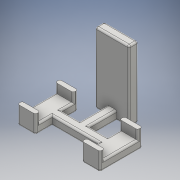
# Autodesk Inventor part: handle
Saved by Autodesk Inventor 2016 (Build 200138000, 138)
## iProperties
Created: 2016-05-24
Part Number: handle
Material: ABS Plastic
Document SubType Name: Modeling
Designer: Hamid Osooli
Density: 1.06 g/cm^3
Appearance: Smooth - White
Mass: 50.8202 g
Surface Area: 188.654 cm^2
Volume: 47.9436 cm^3
Author: Hamid Osooli
Autodesk Inventor part; units mm, degrees
ref_plane "YZ Plane" through (0, 0, 0) normal (1, 0, 0) x (0, 1, 0)
ref_plane "XZ Plane" through (0, 0, 0) normal (0, 1, 0) x (-1, 0, 0)
ref_plane "XY Plane" through (0, 0, 0) normal (0, 0, 1) x (1, 0, 0)
sketch "Sketch1" plane through (0, 0, 0) normal (0, 0, 1) x (1, 0, 0)
  line L0 (42.75, 23) -> (27.25, 23)
  line L1 (25.25, 21) -> (25.25, 20)
  line L2 (27.25, 18) -> (42.75, 18)
  line L3 (44.75, 20) -> (44.75, 21)
  line L4 (-42.75, 23) -> (-27.25, 23)
  line L5 (-25.25, 21) -> (-25.25, 20)
  line L6 (-27.25, 18) -> (-42.75, 18)
  line L7 (-44.75, 20) -> (-44.75, 21)
  line L8 (42.75, -23) -> (27.25, -23)
  line L9 (25.25, -21) -> (25.25, -20)
  line L10 (27.25, -18) -> (42.75, -18)
  line L11 (44.75, -20) -> (44.75, -21)
  line L12 (-42.75, -23) -> (-27.25, -23)
  line L13 (-25.25, -21) -> (-25.25, -20)
  line L14 (-27.25, -18) -> (-42.75, -18)
  line L15 (-44.75, -20) -> (-44.75, -21)
  arc A0 (44.75, 21) -> (42.75, 23) centre (42.75, 21) ccw
  arc A1 (42.75, 18) -> (44.75, 20) centre (42.75, 20) ccw
  arc A2 (25.25, 20) -> (27.25, 18) centre (27.25, 20) ccw
  arc A3 (27.25, 23) -> (25.25, 21) centre (27.25, 21) ccw
  arc A4 (44.75, -20) -> (42.75, -18) centre (42.75, -20) ccw
  arc A5 (42.75, -23) -> (44.75, -21) centre (42.75, -21) ccw
  arc A6 (25.25, -21) -> (27.25, -23) centre (27.25, -21) ccw
  arc A7 (27.25, -18) -> (25.25, -20) centre (27.25, -20) ccw
  arc A8 (-25.25, 21) -> (-27.25, 23) centre (-27.25, 21) ccw
  arc A9 (-27.25, 18) -> (-25.25, 20) centre (-27.25, 20) ccw
  arc A10 (-44.75, 20) -> (-42.75, 18) centre (-42.75, 20) ccw
  arc A11 (-42.75, 23) -> (-44.75, 21) centre (-42.75, 21) ccw
  arc A12 (-25.25, -20) -> (-27.25, -18) centre (-27.25, -20) ccw
  arc A13 (-27.25, -23) -> (-25.25, -21) centre (-27.25, -21) ccw
  arc A14 (-44.75, -21) -> (-42.75, -23) centre (-42.75, -21) ccw
  arc A15 (-42.75, -18) -> (-44.75, -20) centre (-42.75, -20) ccw
  point P0 (25.25, 18)
  point P1 (44.75, 18)
  point P2 (-25.25, 18)
  point P3 (-44.75, 18)
  point P4 (25.25, -18)
  point P5 (44.75, -18)
  point P6 (-25.25, -18)
  point P7 (-44.75, -18)
  dimension "d86" = 19.5
  dimension "d88" = 19.5
  dimension "d90" = 19.5
  dimension "d92" = 19.5
  dimension "d94" = 2
  dimension "d95" = 2
  constraints: 32 end point, 32 point on circle, 32 tangent, 16 centre point, 16 point on line, 14 equal radius, 8 parallel, 4 horizontal, 4 perpendicular
  measures "d86" distance of point (44.75, 18) point (25.25, 18)
  measures "d88" distance of point (-25.25, 18) point (-44.75, 18)
  measures "d90" distance of point (25.25, -18) point (44.75, -18)
  measures "d92" distance of point (-44.75, -18) point (-25.25, -18)
  measures "d94" radius of A0
  measures "d95" radius of A8
extrude "Extrusion1" add sketch "Sketch1" along normal blind 10
sketch "Sketch2" plane through (0, 0, 0) normal (0, 0, 1) x (1, 0, 0)
  line L0 (-42.75, 23) -> (-27.25, 23)
  line L1 (-25.25, 21) -> (-25.25, -21)
  line L2 (-27.25, -23) -> (-42.75, -23)
  line L3 (-44.75, -21) -> (-44.75, 21)
  line L4 (42.75, 23) -> (27.25, 23)
  line L5 (25.25, 21) -> (25.25, -21)
  line L6 (27.25, -23) -> (42.75, -23)
  line L7 (44.75, -21) -> (44.75, 21)
  arc A0 (-42.75, 23) -> (-44.75, 21) centre (-42.75, 21) ccw
  arc A1 (-25.25, 21) -> (-27.25, 23) centre (-27.25, 21) ccw
  arc A2 (-27.25, -23) -> (-25.25, -21) centre (-27.25, -21) ccw
  arc A3 (-44.75, -21) -> (-42.75, -23) centre (-42.75, -21) ccw
  arc A4 (25.25, -21) -> (27.25, -23) centre (27.25, -21) ccw
  arc A5 (42.75, -23) -> (44.75, -21) centre (42.75, -21) ccw
  arc A6 (44.75, 21) -> (42.75, 23) centre (42.75, 21) ccw
  arc A7 (27.25, 23) -> (25.25, 21) centre (27.25, 21) ccw
  point P0 (0, 0)
  point P1 (-25.25, -23)
  point P2 (-25.25, 23)
  point P3 (-44.75, -23)
  point P4 (25.25, -23)
  point P5 (25.25, 23)
  point P6 (44.75, -23)
  dimension "d96" = 19.5
  dimension "d97" = 46
  dimension "d98" = 19.5
  dimension "d99" = 46
  dimension "d100" = 2
  constraints: 16 end point, 16 point on circle, 16 tangent, 12 point on line, 8 centre point, 7 equal radius, 4 parallel, 2 horizontal, 2 perpendicular
  measures "d96" distance of point (-25.25, -23) point (-44.75, -23)
  measures "d97" distance of point (-25.25, 23) point (-25.25, -23)
  measures "d98" distance of point (44.75, -23) point (25.25, -23)
  measures "d99" distance of point (25.25, -23) point (25.25, 23)
  measures "d100" radius of A0
extrude "Extrusion2" add sketch "Sketch2" against normal blind 10
sketch "Sketch9" plane through (25.25, -20, 0) normal (-1, 0, 0) x (0, 0, 1)
  line L0 (0, 0) -> (0, 40) projected
  line L1 (-10, -1) -> (-10, 41) projected
  line L2 (0, 25) -> (-10, 25)
  line L3 (-10, 25) -> (-10, 15)
  line L4 (-10, 15) -> (0, 15)
  line L5 (0, 15) -> (0, 25)
  point P0 (0, 20)
  dimension "d101" = 10
  constraints: 8 end point, 2 parallel, 2 point on line, 1 horizontal, 1 perpendicular
  measures "d101" distance of L3.end L2.end
extrude "Extrusion9" add sketch "Sketch9" along normal up to next
sketch "Sketch12" plane through (0, 0, -10) normal (0, 0, -1) x (-1, 0, 0)
  line L0 (18.5, 35) -> (-18.5, 35)
  line L1 (-18.5, 35) -> (-18.5, 45)
  line L2 (-18.5, 45) -> (18.5, 45)
  line L3 (18.5, 45) -> (18.5, 35)
  point P0 (0, 0)
  dimension "d108" = 37
  dimension "d109" = 10
  constraints: 8 end point, 2 parallel, 1 horizontal, 1 perpendicular
  measures "d108" distance of L1.end L2.end
  measures "d109" distance of L0.end L1.end
extrude "Extrusion11" add sketch "Sketch12" against normal blind 77
sketch "Sketch14" plane through (-18.5, 45, -10) normal (0, 1, 0) x (1, 0, 0)
  line L0 (6.75, -5) -> (30.25, -5)
  line L1 (32.25, -7) -> (32.25, -70)
  line L2 (30.25, -72) -> (6.75, -72)
  line L3 (4.75, -70) -> (4.75, -7)
  arc A0 (6.75, -5) -> (4.75, -7) centre (6.75, -7) ccw
  arc A1 (32.25, -7) -> (30.25, -5) centre (30.25, -7) ccw
  arc A2 (30.25, -72) -> (32.25, -70) centre (30.25, -70) ccw
  arc A3 (4.75, -70) -> (6.75, -72) centre (6.75, -70) ccw
  point P0 (32.25, -72)
  point P1 (32.25, -5)
  point P2 (4.75, -72)
  dimension "d112" = 27.5
  dimension "d113" = 67
  dimension "d114" = 2
  constraints: 8 end point, 8 point on circle, 8 tangent, 6 point on line, 4 centre point, 3 equal radius, 2 parallel, 1 horizontal, 1 perpendicular
  measures "d112" distance of point (32.25, -72) point (4.75, -72)
  measures "d113" distance of point (32.25, -5) point (32.25, -72)
  measures "d114" radius of A0
extrude "Extrusion12" cut sketch "Sketch14" against normal blind 5
sketch "Sketch15" plane through (-18.5, 40, -10) normal (0, 1, 0) x (1, 0, 0)
  circle A0 centre (9.5, -8.5) radius 1.75
  circle A1 centre (27.5, -8.5) radius 1.75
  circle A2 centre (27.5, -68.5) radius 1.75
  circle A3 centre (9.5, -68.5) radius 1.75
  point P0 (18.5, -10)
  dimension "d125" = 3.5
  dimension "d126" = 3.5
  dimension "d127" = 3.5
  dimension "d128" = 3.5
  constraints: 4 centre point
  measures "d125" diameter of A0
  measures "d126" diameter of A1
  measures "d127" diameter of A2
  measures "d128" diameter of A3
extrude "Extrusion13" add sketch "Sketch15" along normal blind 5
sketch "Sketch17" plane through (25.25, 5, 0) normal (0, 1, 0) x (1, 0, 0)
  line L0 (0, 0) -> (-50.5, 0) projected
  line L1 (-30.25, 0) -> (-20.25, 0)
  line L2 (-20.25, 0) -> (-20.25, 10)
  line L3 (-20.25, 10) -> (-30.25, 10)
  line L4 (-30.25, 10) -> (-30.25, 0)
  point P0 (-25.25, 0)
  dimension "d134" = 10
  dimension "d135" = 10
  constraints: 8 end point, 2 parallel, 1 horizontal, 1 perpendicular, 1 point on line
  measures "d134" distance of L3.end L2.end
  measures "d135" distance of L2.end L1.end
extrude "Extrusion15" add sketch "Sketch17" along normal up to next
sketch "Sketch19" plane through (-18.5, 45, -10) normal (0, 1, 0) x (1, 0, 0)
  line L0 (23.5, 0) -> (23.5, -10) projected
  line L1 (13.5, -10) -> (13.5, 0) projected
  line L2 (23.5, -5) -> (13.5, -5)
  line L3 (13.5, -5) -> (13.5, 0)
  line L4 (13.5, 0) -> (23.5, 0)
  line L5 (23.5, 0) -> (23.5, -5)
  point P0 (18.5, -10)
  dimension "d138" = 10
  constraints: 8 end point, 2 parallel, 1 horizontal, 1 midpoint, 1 perpendicular
  measures "d138" distance of L1.end L4.end
extrude "Extrusion16" cut sketch "Sketch19" against normal blind 5
fillet "Fillet5" radius 2 14 edges at (18.5, 45, 28.5) (11.75, 45, -10) (11.75, 35, -10) (18.5, 40, -10) (-11.75, 45, -10) (-11.75, 35, -10) (-18.5, 40, -10) (-18.5, 45, 28.5) (-18.5, 35, 28.5) (-18.5, 40, 67) (0, 35, 67) (18.5, 40, 67) (0, 45, 67) (18.5, 35, 28.5)
fillet "Fillet6" radius 2 24 edges at (-25.8358, 22.4142, -10) (-35, 23, -10) (-44.1642, 22.4142, -10) (-44.75, 0, -10) (-44.1642, -22.4142, -10) (-35, -23, -10) (-25.8358, -22.4142, -10) (-25.25, -13, -10) (-25.25, 13, -10) (-44.75, 0, 0) (-25.25, -12.5, 0) (-25.25, 12.5, 0) (25.25, 12.5, 0) (25.25, -12.5, 0) (44.75, 0, 0) (44.1642, -22.4142, -10) (35, -23, -10) (25.8358, -22.4142, -10) (25.25, -13, -10) (44.1642, 22.4142, -10) (35, 23, -10) (25.8358, 22.4142, -10) (25.25, 13, -10) (44.75, 0, -10)
fillet "Fillet7" radius 2 14 edges at (-26.25, 5, 0) (26.25, 5, 0) (-26.25, -5, 0) (26.25, -5, 0) (5, 20, 0) (-5, 20, 0) (5, 36, -10) (5, 20, -10) (26.25, 5, -10) (-26.25, 5, -10) (-5, 36, -10) (-5, 20, -10) (26.25, -5, -10) (-26.25, -5, -10)
body "Solid1"
